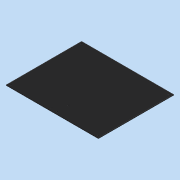
# Autodesk Inventor part: FrameLeftSide
Saved by Autodesk Inventor 2016 (Build 200138000, 138)
## iProperties
Created: 2016-08-20
Part Number: FrameLeftSide
Material: Dibond
Document SubType Name: Modeling
Designer: Sam
Density: 1 g/cm^3
Appearance: Generic
Author: Sam
Autodesk Inventor part; units mm, degrees
ref_plane "YZ Plane" through (0, 0, 0) normal (1, 0, 0) x (0, 1, 0)
ref_plane "XZ Plane" through (0, 0, 0) normal (0, 1, 0) x (-1, 0, 0)
ref_plane "XY Plane" through (0, 0, 0) normal (0, 0, 1) x (1, 0, 0)
sketch "Sketch1" plane through (0, 0, 0) normal (0, 0, 1) x (1, 0, 0)
  line L0 (0, 0) -> (440, 0)
  line L1 (440, 0) -> (440, 360)
  line L2 (440, 360) -> (0, 360)
  line L3 (0, 360) -> (0, 0)
  dimension "d0" = 440
  dimension "d1" = 360
  constraints: 8 end point, 2 parallel, 1 horizontal, 1 perpendicular
  measures "d0" distance of L2.end L1.end
  measures "d1" distance of L1.end L0.end
extrude "Extrusion1" add sketch "Sketch1" along normal blind 3
hole "Hole1" at (12, 12, 3) direction (0, 0, -1) diameter 4 end through all
hole "Hole2" at (428, 12, 3) direction (0, 0, -1) diameter 4 end through all
hole "Hole3" at (428, 348, 3) direction (0, 0, -1) diameter 4 end through all
hole "Hole4" at (12, 348, 3) direction (0, 0, -1) diameter 4 end through all
hole "Hole5" at (233.5, 12, 0) direction (0, 0, 1) diameter 4 end through all
hole "Hole6" at (206.5, 12, 0) direction (0, 0, 1) diameter 4 end through all
hole "Hole7" at (233.5, 63, 0) direction (0, 0, 1) diameter 4 end through all
hole "Hole8" at (233.5, 348, 3) direction (0, 0, -1) diameter 4 end through all
hole "Hole9" at (206.5, 348, 3) direction (0, 0, -1) diameter 4 end through all
body "Solid1"
